Autodesk Fusion 360 part; units mm, degrees
(part 28 of 40)
  line L5956 (42.6094, 50.6358) -> (42.657, 50.79) construction
  line L5957 (42.657, 50.79) -> (42.7037, 50.9447) construction
  line L5958 (42.7037, 50.9447) -> (42.7495, 51.0999) construction
  line L5959 (42.7495, 51.0999) -> (42.7945, 51.2556) construction
  line L5960 (42.7945, 51.2556) -> (42.8386, 51.4118) construction
  line L5961 (42.8386, 51.4118) -> (42.8818, 51.5684) construction
  line L5962 (42.8818, 51.5684) -> (42.9241, 51.7255) construction
  line L5963 (42.9241, 51.7255) -> (42.9656, 51.883) construction
  line L5964 (42.9656, 51.883) -> (43.0063, 52.0409) construction
  line L5965 (43.0063, 52.0409) -> (43.0461, 52.1993) construction
  line L5966 (43.0461, 52.1993) -> (43.085, 52.3581) construction
  line L5967 (43.085, 52.3581) -> (43.1231, 52.5173) construction
  line L5968 (43.1231, 52.5173) -> (43.1604, 52.6769) construction
  line L5969 (43.1604, 52.6769) -> (43.1969, 52.8369) construction
  line L5970 (43.1969, 52.8369) -> (43.2326, 52.9973) construction
  line L5971 (43.2326, 52.9973) -> (43.2674, 53.1581) construction
  line L5972 (43.2674, 53.1581) -> (43.3015, 53.3193) construction
  line L5973 (43.3015, 53.3193) -> (43.3347, 53.4809) construction
  line L5974 (43.3347, 53.4809) -> (43.3672, 53.6428) construction
  line L5975 (43.3672, 53.6428) -> (43.3988, 53.8051) construction
  line L5976 (43.3988, 53.8051) -> (43.4297, 53.9677) construction
  line L5977 (43.4297, 53.9677) -> (43.4597, 54.1307) construction
  line L5978 (43.4597, 54.1307) -> (43.489, 54.294) construction
  line L5979 (43.489, 54.294) -> (43.5175, 54.4577) construction
  line L5980 (43.5175, 54.4577) -> (43.5453, 54.6217) construction
  line L5981 (43.5453, 54.6217) -> (43.5723, 54.7861) construction
  line L5982 (43.5723, 54.7861) -> (43.5984, 54.9508) construction
  line L5983 (43.5984, 54.9508) -> (43.6239, 55.1158) construction
  line L5984 (43.6239, 55.1158) -> (43.6486, 55.2811) construction
  line L5985 (43.6486, 55.2811) -> (43.6725, 55.4467) construction
  line L5986 (43.6725, 55.4467) -> (43.6956, 55.6126) construction
  line L5987 (43.6956, 55.6126) -> (43.718, 55.7789) construction
  line L5988 (43.718, 55.7789) -> (43.7397, 55.9454) construction
  line L5989 (43.7397, 55.9454) -> (43.7606, 56.1122) construction
  line L5990 (43.7606, 56.1122) -> (43.7767, 56.2459) construction
  line L5991 (43.7767, 56.2459) -> (43.7885, 56.3463) construction
  line L5992 (43.7885, 56.3463) -> (43.7962, 56.4133) construction
  line L5993 (43.7962, 56.4133) -> (43.8, 56.4469) construction
  arc A159 (-24.5301, 51.9354) -> (-27.5982, 50.3721) centre (0, 0) ccw
  arc A160 (-41.8132, -39.3784) -> (-39.3784, -41.8132) centre (0, 0) ccw
  line L5994 (-54.5366, 23.5481) -> (-56.0345, 24.1948)
  line L5995 (-57.9623, -13.005) -> (-59.5542, -13.3622)
  line L5996 (-44.5906, 39.2483) -> (-45.8153, 40.3263)
  line L5997 (13.005, 57.9623) -> (13.3622, 59.5542)
  line L5998 (51.1066, 30.2798) -> (52.5103, 31.1115)
  line L5999 (30.2798, -51.1066) -> (31.1115, -52.5103)
  arc A161 (41.8132, 39.3784) -> (39.3784, 41.8132) centre (0, 0) ccw
  line L6000 (157.5954, 173.5481) -> (156.0975, 174.1948)
  line L6001 (266.6686, 173.5481) -> (268.1665, 174.1948)
  line L6002 (271.2762, 155.5428) -> (272.9005, 155.6951)
  line L6003 (206.5892, 209.1442) -> (206.4369, 210.7685)
  line L6004 (199.127, 207.9623) -> (198.7698, 209.5542)
  line L6005 (251.3803, 194.5906) -> (252.4583, 195.8153)
  line L6006 (188.5839, 95.4634) -> (187.9372, 93.9655)
  arc A162 (157.5954, 173.5481) -> (160.1966, 174.5301) centre (158.3882, 175.3842) ccw
  arc A163 (160.1966, 125.4699) -> (157.5954, 126.4519) centre (158.3882, 124.6158) ccw
  arc A164 (251.5104, 108.1868) -> (251.3803, 105.4094) centre (252.8816, 106.7308) ccw
  arc A165 (262.5041, 122.4018) -> (263.2386, 119.7202) centre (264.2581, 121.4408) ccw
  spline S80 degree 5 poles (152.5778, 136.6378) (152.5477, 136.631) (152.4876, 136.6167) (152.3982, 136.5929) (152.2803, 136.5565) (152.1347, 136.5049) (151.9904, 136.4489) (151.8468, 136.3901) (151.7037, 136.3299) (151.5609, 136.2687) (151.4184, 136.2065) (151.2763, 136.1429) (151.1349, 136.0774) (150.9941, 136.0098) (150.8541, 135.94) (150.7147, 135.8684) (150.5759, 135.795) (150.4376, 135.7203) (150.2998, 135.6443) (150.1623, 135.5673) (150.0253, 135.4891) (149.8888, 135.4096) (149.7528, 135.3289) (149.6172, 135.247) (149.4822, 135.1637) (149.3477, 135.0792) (149.2136, 134.9936) (149.08, 134.9068) (148.9468, 134.819) (148.814, 134.7302) (148.6817, 134.6403) (148.5499, 134.5494) (148.4185, 134.4575) (148.2875, 134.3646) (148.157, 134.2707) (148.027, 134.1758) (147.8974, 134.08) (147.7682, 133.9832) (147.6394, 133.8854) (147.5111, 133.7868) (147.3832, 133.6873) (147.2558, 133.5869) (147.1288, 133.4856) (147.0022, 133.3834) (146.876, 133.2804) (146.7503, 133.1765) (146.625, 133.0717) (146.5002, 132.9662) (146.3758, 132.8598) (146.2518, 132.7526) (146.1282, 132.6445) (146.0051, 132.5357) (145.8823, 132.4261) (145.7601, 132.3158) (145.6382, 132.2046) (145.5168, 132.0927) (145.3958, 131.98) (145.2752, 131.8665) (145.1551, 131.7523) (145.0354, 131.6374) (144.9161, 131.5218) (144.7973, 131.4054) (144.6789, 131.2882) (144.5609, 131.1704) (144.4433, 131.0519) (144.3262, 130.9326) (144.2095, 130.8127) (144.0932, 130.6921) (143.9774, 130.5707) (143.862, 130.4488) (143.747, 130.3261) (143.6553, 130.2274) (143.5868, 130.1531) (143.5412, 130.1034) (143.5184, 130.0785) knots 0 0 0 0 0 0 0.01428571 0.02857143 0.04285714 0.05714286 0.07142857 0.08571429 0.1 0.11428571 0.12857143 0.14285714 0.15714286 0.17142857 0.18571429 0.2 0.21428571 0.22857143 0.24285714 0.25714286 0.27142857 0.28571429 0.3 0.31428571 0.32857143 0.34285714 0.35714286 0.37142857 0.38571429 0.4 0.41428571 0.42857143 0.44285714 0.45714286 0.47142857 0.48571429 0.5 0.51428571 0.52857143 0.54285714 0.55714286 0.57142857 0.58571429 0.6 0.61428571 0.62857143 0.64285714 0.65714286 0.67142857 0.68571429 0.7 0.71428571 0.72857143 0.74285714 0.75714286 0.77142857 0.78571429 0.8 0.81428571 0.82857143 0.84285714 0.85714286 0.87142857 0.88571429 0.9 0.91428571 0.92857143 0.94285714 0.95714286 0.97142857 0.98571429 1 1 1 1 1 1
  line L6007 (152.5778, 136.6378) -> (152.5477, 136.631) construction
  line L6008 (152.5477, 136.631) -> (152.4876, 136.6167) construction
  line L6009 (152.4876, 136.6167) -> (152.3982, 136.5929) construction
  line L6010 (152.3982, 136.5929) -> (152.2803, 136.5565) construction
  line L6011 (152.2803, 136.5565) -> (152.1347, 136.5049) construction
  line L6012 (152.1347, 136.5049) -> (151.9904, 136.4489) construction
  line L6013 (151.9904, 136.4489) -> (151.8468, 136.3901) construction
  line L6014 (151.8468, 136.3901) -> (151.7037, 136.3299) construction
  line L6015 (151.7037, 136.3299) -> (151.5609, 136.2687) construction
  line L6016 (151.5609, 136.2687) -> (151.4184, 136.2065) construction
  line L6017 (151.4184, 136.2065) -> (151.2763, 136.1429) construction
  line L6018 (151.2763, 136.1429) -> (151.1349, 136.0774) construction
  line L6019 (151.1349, 136.0774) -> (150.9941, 136.0098) construction
  line L6020 (150.9941, 136.0098) -> (150.8541, 135.94) construction
  line L6021 (150.8541, 135.94) -> (150.7147, 135.8684) construction
  line L6022 (150.7147, 135.8684) -> (150.5759, 135.795) construction
  line L6023 (150.5759, 135.795) -> (150.4376, 135.7203) construction
  line L6024 (150.4376, 135.7203) -> (150.2998, 135.6443) construction
  line L6025 (150.2998, 135.6443) -> (150.1623, 135.5673) construction
  line L6026 (150.1623, 135.5673) -> (150.0253, 135.4891) construction
  line L6027 (150.0253, 135.4891) -> (149.8888, 135.4096) construction
  line L6028 (149.8888, 135.4096) -> (149.7528, 135.3289) construction
  line L6029 (149.7528, 135.3289) -> (149.6172, 135.247) construction
  line L6030 (149.6172, 135.247) -> (149.4822, 135.1637) construction
  line L6031 (149.4822, 135.1637) -> (149.3477, 135.0792) construction
  line L6032 (149.3477, 135.0792) -> (149.2136, 134.9936) construction
  line L6033 (149.2136, 134.9936) -> (149.08, 134.9068) construction
  line L6034 (149.08, 134.9068) -> (148.9468, 134.819) construction
  line L6035 (148.9468, 134.819) -> (148.814, 134.7302) construction
  line L6036 (148.814, 134.7302) -> (148.6817, 134.6403) construction
  line L6037 (148.6817, 134.6403) -> (148.5499, 134.5494) construction
  line L6038 (148.5499, 134.5494) -> (148.4185, 134.4575) construction
  line L6039 (148.4185, 134.4575) -> (148.2875, 134.3646) construction
  line L6040 (148.2875, 134.3646) -> (148.157, 134.2707) construction
  line L6041 (148.157, 134.2707) -> (148.027, 134.1758) construction
  line L6042 (148.027, 134.1758) -> (147.8974, 134.08) construction
  line L6043 (147.8974, 134.08) -> (147.7682, 133.9832) construction
  line L6044 (147.7682, 133.9832) -> (147.6394, 133.8854) construction
  line L6045 (147.6394, 133.8854) -> (147.5111, 133.7868) construction
  line L6046 (147.5111, 133.7868) -> (147.3832, 133.6873) construction
  line L6047 (147.3832, 133.6873) -> (147.2558, 133.5869) construction
  line L6048 (147.2558, 133.5869) -> (147.1288, 133.4856) construction
  line L6049 (147.1288, 133.4856) -> (147.0022, 133.3834) construction
  line L6050 (147.0022, 133.3834) -> (146.876, 133.2804) construction
  line L6051 (146.876, 133.2804) -> (146.7503, 133.1765) construction
  line L6052 (146.7503, 133.1765) -> (146.625, 133.0717) construction
  line L6053 (146.625, 133.0717) -> (146.5002, 132.9662) construction
  line L6054 (146.5002, 132.9662) -> (146.3758, 132.8598) construction
  line L6055 (146.3758, 132.8598) -> (146.2518, 132.7526) construction
  line L6056 (146.2518, 132.7526) -> (146.1282, 132.6445) construction
  line L6057 (146.1282, 132.6445) -> (146.0051, 132.5357) construction
  line L6058 (146.0051, 132.5357) -> (145.8823, 132.4261) construction
  line L6059 (145.8823, 132.4261) -> (145.7601, 132.3158) construction
  line L6060 (145.7601, 132.3158) -> (145.6382, 132.2046) construction
  line L6061 (145.6382, 132.2046) -> (145.5168, 132.0927) construction
  line L6062 (145.5168, 132.0927) -> (145.3958, 131.98) construction
  line L6063 (145.3958, 131.98) -> (145.2752, 131.8665) construction
  line L6064 (145.2752, 131.8665) -> (145.1551, 131.7523) construction
  line L6065 (145.1551, 131.7523) -> (145.0354, 131.6374) construction
  line L6066 (145.0354, 131.6374) -> (144.9161, 131.5218) construction
  line L6067 (144.9161, 131.5218) -> (144.7973, 131.4054) construction
  line L6068 (144.7973, 131.4054) -> (144.6789, 131.2882) construction
  line L6069 (144.6789, 131.2882) -> (144.5609, 131.1704) construction
  line L6070 (144.5609, 131.1704) -> (144.4433, 131.0519) construction
  line L6071 (144.4433, 131.0519) -> (144.3262, 130.9326) construction
  line L6072 (144.3262, 130.9326) -> (144.2095, 130.8127) construction
  line L6073 (144.2095, 130.8127) -> (144.0932, 130.6921) construction
  line L6074 (144.0932, 130.6921) -> (143.9774, 130.5707) construction
  line L6075 (143.9774, 130.5707) -> (143.862, 130.4488) construction
  line L6076 (143.862, 130.4488) -> (143.747, 130.3261) construction
  line L6077 (143.747, 130.3261) -> (143.6553, 130.2274) construction
  line L6078 (143.6553, 130.2274) -> (143.5868, 130.1531) construction
  line L6079 (143.5868, 130.1531) -> (143.5412, 130.1034) construction
  line L6080 (143.5412, 130.1034) -> (143.5184, 130.0785) construction
  arc A166 (155.6851, 193.8) -> (153.0327, 190.1492) centre (212.132, 150) ccw
  spline S81 degree 5 poles (181.0205, 202.5103) (181.0048, 202.5368) (180.9726, 202.5895) (180.9223, 202.6672) (180.8513, 202.7681) (180.7572, 202.8906) (180.6593, 203.0106) (180.5591, 203.1289) (180.4576, 203.2464) (180.3553, 203.3634) (180.252, 203.4797) (180.1476, 203.5951) (180.0417, 203.7094) (179.9339, 203.8224) (179.8243, 203.934) (179.713, 204.0444) (179.6004, 204.1537) (179.4865, 204.2622) (179.3717, 204.3698) (179.256, 204.4767) (179.1393, 204.5828) (179.0215, 204.6881) (178.9028, 204.7926) (178.7829, 204.8961) (178.662, 204.9988) (178.5401, 205.1007) (178.4172, 205.2017) (178.2934, 205.302) (178.1687, 205.4015) (178.0432, 205.5003) (177.9169, 205.5984) (177.7897, 205.6957) (177.6617, 205.7923) (177.5329, 205.8881) (177.4032, 205.9832) (177.2728, 206.0776) (177.1415, 206.1712) (177.0096, 206.2642) (176.8768, 206.3564) (176.7434, 206.448) (176.6092, 206.5388) (176.4743, 206.629) (176.3387, 206.7185) (176.2025, 206.8073) (176.0655, 206.8955) (175.9278, 206.9829) (175.7895, 207.0697) (175.6505, 207.1558) (175.5109, 207.2413) (175.3706, 207.3261) (175.2297, 207.4102) (175.0882, 207.4937) (174.946, 207.5765) (174.8032, 207.6587) (174.6599, 207.7403) (174.5159, 207.8212) (174.3713, 207.9014) (174.2262, 207.981) (174.0805, 208.06) (173.9342, 208.1383) (173.7873, 208.216) (173.6399, 208.2931) (173.4919, 208.3695) (173.3434, 208.4453) (173.1943, 208.5205) (173.0447, 208.595) (172.8946, 208.669) (172.7439, 208.7423) (172.5927, 208.8149) (172.4411, 208.887) (172.2889, 208.9584) (172.1667, 209.0151) (172.0748, 209.0573) (172.0135, 209.0853) (171.9828, 209.0993) knots 0 0 0 0 0 0 0.01428571 0.02857143 0.04285714 0.05714286 0.07142857 0.08571429 0.1 0.11428571 0.12857143 0.14285714 0.15714286 0.17142857 0.18571429 0.2 0.21428571 0.22857143 0.24285714 0.25714286 0.27142857 0.28571429 0.3 0.31428571 0.32857143 0.34285714 0.35714286 0.37142857 0.38571429 0.4 0.41428571 0.42857143 0.44285714 0.45714286 0.47142857 0.48571429 0.5 0.51428571 0.52857143 0.54285714 0.55714286 0.57142857 0.58571429 0.6 0.61428571 0.62857143 0.64285714 0.65714286 0.67142857 0.68571429 0.7 0.71428571 0.72857143 0.74285714 0.75714286 0.77142857 0.78571429 0.8 0.81428571 0.82857143 0.84285714 0.85714286 0.87142857 0.88571429 0.9 0.91428571 0.92857143 0.94285714 0.95714286 0.97142857 0.98571429 1 1 1 1 1 1
  line L6081 (181.0205, 202.5103) -> (181.0048, 202.5368) construction
  line L6082 (181.0048, 202.5368) -> (180.9726, 202.5895) construction
  line L6083 (180.9726, 202.5895) -> (180.9223, 202.6672) construction
  line L6084 (180.9223, 202.6672) -> (180.8513, 202.7681) construction
  line L6085 (180.8513, 202.7681) -> (180.7572, 202.8906) construction
  line L6086 (180.7572, 202.8906) -> (180.6593, 203.0106) construction
  line L6087 (180.6593, 203.0106) -> (180.5591, 203.1289) construction
  line L6088 (180.5591, 203.1289) -> (180.4576, 203.2464) construction
  line L6089 (180.4576, 203.2464) -> (180.3553, 203.3634) construction
  line L6090 (180.3553, 203.3634) -> (180.252, 203.4797) construction
  line L6091 (180.252, 203.4797) -> (180.1476, 203.5951) construction
  line L6092 (180.1476, 203.5951) -> (180.0417, 203.7094) construction
  line L6093 (180.0417, 203.7094) -> (179.9339, 203.8224) construction
  line L6094 (179.9339, 203.8224) -> (179.8243, 203.934) construction
  line L6095 (179.8243, 203.934) -> (179.713, 204.0444) construction
  line L6096 (179.713, 204.0444) -> (179.6004, 204.1537) construction
  line L6097 (179.6004, 204.1537) -> (179.4865, 204.2622) construction
  line L6098 (179.4865, 204.2622) -> (179.3717, 204.3698) construction
  line L6099 (179.3717, 204.3698) -> (179.256, 204.4767) construction
  line L6100 (179.256, 204.4767) -> (179.1393, 204.5828) construction
  line L6101 (179.1393, 204.5828) -> (179.0215, 204.6881) construction
  line L6102 (179.0215, 204.6881) -> (178.9028, 204.7926) construction
  line L6103 (178.9028, 204.7926) -> (178.7829, 204.8961) construction
  line L6104 (178.7829, 204.8961) -> (178.662, 204.9988) construction
  line L6105 (178.662, 204.9988) -> (178.5401, 205.1007) construction
  line L6106 (178.5401, 205.1007) -> (178.4172, 205.2017) construction
  line L6107 (178.4172, 205.2017) -> (178.2934, 205.302) construction
  line L6108 (178.2934, 205.302) -> (178.1687, 205.4015) construction
  line L6109 (178.1687, 205.4015) -> (178.0432, 205.5003) construction
  line L6110 (178.0432, 205.5003) -> (177.9169, 205.5984) construction
  line L6111 (177.9169, 205.5984) -> (177.7897, 205.6957) construction
  line L6112 (177.7897, 205.6957) -> (177.6617, 205.7923) construction
  line L6113 (177.6617, 205.7923) -> (177.5329, 205.8881) construction
  line L6114 (177.5329, 205.8881) -> (177.4032, 205.9832) construction
  line L6115 (177.4032, 205.9832) -> (177.2728, 206.0776) construction
  line L6116 (177.2728, 206.0776) -> (177.1415, 206.1712) construction
  line L6117 (177.1415, 206.1712) -> (177.0096, 206.2642) construction
  line L6118 (177.0096, 206.2642) -> (176.8768, 206.3564) construction
  line L6119 (176.8768, 206.3564) -> (176.7434, 206.448) construction
  line L6120 (176.7434, 206.448) -> (176.6092, 206.5388) construction
  line L6121 (176.6092, 206.5388) -> (176.4743, 206.629) construction
  line L6122 (176.4743, 206.629) -> (176.3387, 206.7185) construction
  line L6123 (176.3387, 206.7185) -> (176.2025, 206.8073) construction
  line L6124 (176.2025, 206.8073) -> (176.0655, 206.8955) construction
  line L6125 (176.0655, 206.8955) -> (175.9278, 206.9829) construction
  line L6126 (175.9278, 206.9829) -> (175.7895, 207.0697) construction
  line L6127 (175.7895, 207.0697) -> (175.6505, 207.1558) construction
  line L6128 (175.6505, 207.1558) -> (175.5109, 207.2413) construction
  line L6129 (175.5109, 207.2413) -> (175.3706, 207.3261) construction
  line L6130 (175.3706, 207.3261) -> (175.2297, 207.4102) construction
  line L6131 (175.2297, 207.4102) -> (175.0882, 207.4937) construction
  line L6132 (175.0882, 207.4937) -> (174.946, 207.5765) construction
  line L6133 (174.946, 207.5765) -> (174.8032, 207.6587) construction
  line L6134 (174.8032, 207.6587) -> (174.6599, 207.7403) construction
  line L6135 (174.6599, 207.7403) -> (174.5159, 207.8212) construction
  line L6136 (174.5159, 207.8212) -> (174.3713, 207.9014) construction
  line L6137 (174.3713, 207.9014) -> (174.2262, 207.981) construction
  line L6138 (174.2262, 207.981) -> (174.0805, 208.06) construction
  line L6139 (174.0805, 208.06) -> (173.9342, 208.1383) construction
  line L6140 (173.9342, 208.1383) -> (173.7873, 208.216) construction
  line L6141 (173.7873, 208.216) -> (173.6399, 208.2931) construction
  line L6142 (173.6399, 208.2931) -> (173.4919, 208.3695) construction
  line L6143 (173.4919, 208.3695) -> (173.3434, 208.4453) construction
  line L6144 (173.3434, 208.4453) -> (173.1943, 208.5205) construction
  line L6145 (173.1943, 208.5205) -> (173.0447, 208.595) construction
  line L6146 (173.0447, 208.595) -> (172.8946, 208.669) construction
  line L6147 (172.8946, 208.669) -> (172.7439, 208.7423) construction
  line L6148 (172.7439, 208.7423) -> (172.5927, 208.8149) construction
  line L6149 (172.5927, 208.8149) -> (172.4411, 208.887) construction
  line L6150 (172.4411, 208.887) -> (172.2889, 208.9584) construction
  line L6151 (172.2889, 208.9584) -> (172.1667, 209.0151) construction
  line L6152 (172.1667, 209.0151) -> (172.0748, 209.0573) construction
  line L6153 (172.0748, 209.0573) -> (172.0135, 209.0853) construction
  line L6154 (172.0135, 209.0853) -> (171.9828, 209.0993) construction
  spline S82 degree 5 poles (198.7698, 209.5542) (198.763, 209.5843) (198.7487, 209.6444) (198.7249, 209.7338) (198.6885, 209.8517) (198.6369, 209.9973) (198.5809, 210.1416) (198.5221, 210.2852) (198.4619, 210.4283) (198.4007, 210.5711) (198.3385, 210.7136) (198.2749, 210.8557) (198.2094, 210.9971) (198.1418, 211.1379) (198.072, 211.2779) (198.0004, 211.4173) (197.927, 211.5561) (197.8523, 211.6944) (197.7763, 211.8322) (197.6993, 211.9697) (197.6211, 212.1067) (197.5416, 212.2432) (197.4609, 212.3792) (197.379, 212.5148) (197.2957, 212.6498) (197.2112, 212.7843) (197.1256, 212.9184) (197.0388, 213.052) (196.951, 213.1852) (196.8622, 213.318) (196.7723, 213.4503) (196.6814, 213.5821) (196.5895, 213.7135) (196.4966, 213.8445) (196.4027, 213.975) (196.3078, 214.105) (196.212, 214.2346) (196.1152, 214.3638) (196.0174, 214.4926) (195.9188, 214.6209) (195.8193, 214.7488) (195.7189, 214.8762) (195.6176, 215.0032) (195.5154, 215.1298) (195.4124, 215.256) (195.3085, 215.3817) (195.2037, 215.507) (195.0982, 215.6318) (194.9918, 215.7562) (194.8846, 215.8802) (194.7765, 216.0038) (194.6677, 216.1269) (194.5581, 216.2497) (194.4478, 216.3719) (194.3366, 216.4938) (194.2247, 216.6152) (194.112, 216.7362) (193.9985, 216.8568) (193.8843, 216.9769) (193.7694, 217.0966) (193.6538, 217.2159) (193.5374, 217.3347) (193.4202, 217.4531) (193.3024, 217.5711) (193.1839, 217.6887) (193.0646, 217.8058) (192.9447, 217.9225) (192.8241, 218.0388) (192.7027, 218.1546) (192.5808, 218.27) (192.4581, 218.385) (192.3594, 218.4767) (192.2851, 218.5452) (192.2354, 218.5908) (192.2105, 218.6136) knots 0 0 0 0 0 0 0.01428571 0.02857143 0.04285714 0.05714286 0.07142857 0.08571429 0.1 0.11428571 0.12857143 0.14285714 0.15714286 0.17142857 0.18571429 0.2 0.21428571 0.22857143 0.24285714 0.25714286 0.27142857 0.28571429 0.3 0.31428571 0.32857143 0.34285714 0.35714286 0.37142857 0.38571429 0.4 0.41428571 0.42857143 0.44285714 0.45714286 0.47142857 0.48571429 0.5 0.51428571 0.52857143 0.54285714 0.55714286 0.57142857 0.58571429 0.6 0.61428571 0.62857143 0.64285714 0.65714286 0.67142857 0.68571429 0.7 0.71428571 0.72857143 0.74285714 0.75714286 0.77142857 0.78571429 0.8 0.81428571 0.82857143 0.84285714 0.85714286 0.87142857 0.88571429 0.9 0.91428571 0.92857143 0.94285714 0.95714286 0.97142857 0.98571429 1 1 1 1 1 1
  line L6155 (198.7698, 209.5542) -> (198.763, 209.5843) construction
  line L6156 (198.763, 209.5843) -> (198.7487, 209.6444) construction
  line L6157 (198.7487, 209.6444) -> (198.7249, 209.7338) construction
  line L6158 (198.7249, 209.7338) -> (198.6885, 209.8517) construction
  line L6159 (198.6885, 209.8517) -> (198.6369, 209.9973) construction
  line L6160 (198.6369, 209.9973) -> (198.5809, 210.1416) construction
  line L6161 (198.5809, 210.1416) -> (198.5221, 210.2852) construction
  line L6162 (198.5221, 210.2852) -> (198.4619, 210.4283) construction
  line L6163 (198.4619, 210.4283) -> (198.4007, 210.5711) construction
  line L6164 (198.4007, 210.5711) -> (198.3385, 210.7136) construction
  line L6165 (198.3385, 210.7136) -> (198.2749, 210.8557) construction
  line L6166 (198.2749, 210.8557) -> (198.2094, 210.9971) construction
  line L6167 (198.2094, 210.9971) -> (198.1418, 211.1379) construction
  line L6168 (198.1418, 211.1379) -> (198.072, 211.2779) construction
  line L6169 (198.072, 211.2779) -> (198.0004, 211.4173) construction
  line L6170 (198.0004, 211.4173) -> (197.927, 211.5561) construction
  line L6171 (197.927, 211.5561) -> (197.8523, 211.6944) construction
  line L6172 (197.8523, 211.6944) -> (197.7763, 211.8322) construction
  line L6173 (197.7763, 211.8322) -> (197.6993, 211.9697) construction
  line L6174 (197.6993, 211.9697) -> (197.6211, 212.1067) construction
  line L6175 (197.6211, 212.1067) -> (197.5416, 212.2432) construction
  line L6176 (197.5416, 212.2432) -> (197.4609, 212.3792) construction
  line L6177 (197.4609, 212.3792) -> (197.379, 212.5148) construction
  line L6178 (197.379, 212.5148) -> (197.2957, 212.6498) construction
  line L6179 (197.2957, 212.6498) -> (197.2112, 212.7843) construction
  line L6180 (197.2112, 212.7843) -> (197.1256, 212.9184) construction
  line L6181 (197.1256, 212.9184) -> (197.0388, 213.052) construction
  line L6182 (197.0388, 213.052) -> (196.951, 213.1852) construction
  line L6183 (196.951, 213.1852) -> (196.8622, 213.318) construction
  line L6184 (196.8622, 213.318) -> (196.7723, 213.4503) construction
  line L6185 (196.7723, 213.4503) -> (196.6814, 213.5821) construction
  line L6186 (196.6814, 213.5821) -> (196.5895, 213.7135) construction
  line L6187 (196.5895, 213.7135) -> (196.4966, 213.8445) construction
  line L6188 (196.4966, 213.8445) -> (196.4027, 213.975) construction
  line L6189 (196.4027, 213.975) -> (196.3078, 214.105) construction
  line L6190 (196.3078, 214.105) -> (196.212, 214.2346) construction
  line L6191 (196.212, 214.2346) -> (196.1152, 214.3638) construction
  line L6192 (196.1152, 214.3638) -> (196.0174, 214.4926) construction
  line L6193 (196.0174, 214.4926) -> (195.9188, 214.6209) construction
  line L6194 (195.9188, 214.6209) -> (195.8193, 214.7488) construction
  line L6195 (195.8193, 214.7488) -> (195.7189, 214.8762) construction
  line L6196 (195.7189, 214.8762) -> (195.6176, 215.0032) construction
  line L6197 (195.6176, 215.0032) -> (195.5154, 215.1298) construction
  line L6198 (195.5154, 215.1298) -> (195.4124, 215.256) construction
  line L6199 (195.4124, 215.256) -> (195.3085, 215.3817) construction
  line L6200 (195.3085, 215.3817) -> (195.2037, 215.507) construction
  line L6201 (195.2037, 215.507) -> (195.0982, 215.6318) construction
  line L6202 (195.0982, 215.6318) -> (194.9918, 215.7562) construction
  line L6203 (194.9918, 215.7562) -> (194.8846, 215.8802) construction
  line L6204 (194.8846, 215.8802) -> (194.7765, 216.0038) construction
  line L6205 (194.7765, 216.0038) -> (194.6677, 216.1269) construction
  line L6206 (194.6677, 216.1269) -> (194.5581, 216.2497) construction
  line L6207 (194.5581, 216.2497) -> (194.4478, 216.3719) construction
  line L6208 (194.4478, 216.3719) -> (194.3366, 216.4938) construction
  line L6209 (194.3366, 216.4938) -> (194.2247, 216.6152) construction
  line L6210 (194.2247, 216.6152) -> (194.112, 216.7362) construction
  line L6211 (194.112, 216.7362) -> (193.9985, 216.8568) construction
  line L6212 (193.9985, 216.8568) -> (193.8843, 216.9769) construction
  line L6213 (193.8843, 216.9769) -> (193.7694, 217.0966) construction
  line L6214 (193.7694, 217.0966) -> (193.6538, 217.2159) construction
  line L6215 (193.6538, 217.2159) -> (193.5374, 217.3347) construction
  line L6216 (193.5374, 217.3347) -> (193.4202, 217.4531) construction
  line L6217 (193.4202, 217.4531) -> (193.3024, 217.5711) construction
  line L6218 (193.3024, 217.5711) -> (193.1839, 217.6887) construction
  line L6219 (193.1839, 217.6887) -> (193.0646, 217.8058) construction
  line L6220 (193.0646, 217.8058) -> (192.9447, 217.9225) construction
  line L6221 (192.9447, 217.9225) -> (192.8241, 218.0388) construction
  line L6222 (192.8241, 218.0388) -> (192.7027, 218.1546) construction
  line L6223 (192.7027, 218.1546) -> (192.5808, 218.27) construction
  line L6224 (192.5808, 218.27) -> (192.4581, 218.385) construction
  line L6225 (192.4581, 218.385) -> (192.3594, 218.4767) construction
  line L6226 (192.3594, 218.4767) -> (192.2851, 218.5452) construction
  line L6227 (192.2851, 218.5452) -> (192.2354, 218.5908) construction
  line L6228 (192.2354, 218.5908) -> (192.2105, 218.6136) construction
  arc A167 (255.932, 206.4469) -> (252.2812, 209.0993) centre (212.132, 150) ccw
  arc A168 (271.2313, 190.1492) -> (268.5789, 193.8) centre (212.132, 150) ccw
  spline S83 degree 5 poles (272.9005, 155.6951) (272.9313, 155.6979) (272.9929, 155.7029) (273.0853, 155.7078) (273.2086, 155.7097) (273.363, 155.7056) (273.5176, 155.6969) (273.6723, 155.6854) (273.827, 155.6723) (273.9818, 155.6583) (274.1365, 155.6431) (274.2913, 155.6265) (274.446, 155.608) (274.6008, 155.5871) (274.7555, 155.5641) (274.9102, 155.539) (275.0649, 155.5121) (275.2195, 155.4838) (275.3741, 155.4542) (275.5286, 155.4233) (275.6831, 155.3913) (275.8375, 155.3579) (275.9918, 155.3232) (276.146, 155.2871) (276.3002, 155.2497) (276.4542, 155.2109) (276.6082, 155.1709) (276.7621, 155.1297) (276.9159, 155.0873) (277.0696, 155.0439) (277.2232, 154.9993) (277.3767, 154.9536) (277.53, 154.9068) (277.6833, 154.8589) (277.8364, 154.8099) (277.9894, 154.7599) (278.1423, 154.7087) (278.2951, 154.6566) (278.4478, 154.6035) (278.6003, 154.5493) (278.7526, 154.4942) (278.9049, 154.438) (279.057, 154.381) (279.209, 154.3229) (279.3608, 154.2639) (279.5124, 154.2039) (279.664, 154.143) (279.8153, 154.0812) (279.9665, 154.0185) (280.1176, 153.9548) (280.2685, 153.8903) (280.4192, 153.8249) (280.5698, 153.7585) (280.7202, 153.6913) (280.8704, 153.6233) (281.0205, 153.5543) (281.1704, 153.4846) (281.3201, 153.4139) (281.4696, 153.3425) (281.619, 153.2701) (281.7682, 153.197) (281.9172, 153.123) (282.066, 153.0482) (282.2146, 152.9726) (282.3631, 152.8962) (282.5113, 152.819) (282.6594, 152.741) (282.8072, 152.6622) (282.9549, 152.5826) (283.1023, 152.5023) (283.2496, 152.4211) (283.3672, 152.3556) (283.4554, 152.3061) (283.5141, 152.2729) (283.5435, 152.2563) knots 0 0 0 0 0 0 0.01428571 0.02857143 0.04285714 0.05714286 0.07142857 0.08571429 0.1 0.11428571 0.12857143 0.14285714 0.15714286 0.17142857 0.18571429 0.2 0.21428571 0.22857143 0.24285714 0.25714286 0.27142857 0.28571429 0.3 0.31428571 0.32857143 0.34285714 0.35714286 0.37142857 0.38571429 0.4 0.41428571 0.42857143 0.44285714 0.45714286 0.47142857 0.48571429 0.5 0.51428571 0.52857143 0.54285714 0.55714286 0.57142857 0.58571429 0.6 0.61428571 0.62857143 0.64285714 0.65714286 0.67142857 0.68571429 0.7 0.71428571 0.72857143 0.74285714 0.75714286 0.77142857 0.78571429 0.8 0.81428571 0.82857143 0.84285714 0.85714286 0.87142857 0.88571429 0.9 0.91428571 0.92857143 0.94285714 0.95714286 0.97142857 0.98571429 1 1 1 1 1 1
  line L6229 (272.9005, 155.6951) -> (272.9313, 155.6979) construction
  line L6230 (272.9313, 155.6979) -> (272.9929, 155.7029) construction
  line L6231 (272.9929, 155.7029) -> (273.0853, 155.7078) construction
  line L6232 (273.0853, 155.7078) -> (273.2086, 155.7097) construction
  line L6233 (273.2086, 155.7097) -> (273.363, 155.7056) construction
  line L6234 (273.363, 155.7056) -> (273.5176, 155.6969) construction
  line L6235 (273.5176, 155.6969) -> (273.6723, 155.6854) construction
  line L6236 (273.6723, 155.6854) -> (273.827, 155.6723) construction
  line L6237 (273.827, 155.6723) -> (273.9818, 155.6583) construction
  line L6238 (273.9818, 155.6583) -> (274.1365, 155.6431) construction
  line L6239 (274.1365, 155.6431) -> (274.2913, 155.6265) construction
  line L6240 (274.2913, 155.6265) -> (274.446, 155.608) construction
  line L6241 (274.446, 155.608) -> (274.6008, 155.5871) construction
  line L6242 (274.6008, 155.5871) -> (274.7555, 155.5641) construction
  line L6243 (274.7555, 155.5641) -> (274.9102, 155.539) construction
  line L6244 (274.9102, 155.539) -> (275.0649, 155.5121) construction
  line L6245 (275.0649, 155.5121) -> (275.2195, 155.4838) construction
  line L6246 (275.2195, 155.4838) -> (275.3741, 155.4542) construction
  line L6247 (275.3741, 155.4542) -> (275.5286, 155.4233) construction
  line L6248 (275.5286, 155.4233) -> (275.6831, 155.3913) construction
  line L6249 (275.6831, 155.3913) -> (275.8375, 155.3579) construction
  line L6250 (275.8375, 155.3579) -> (275.9918, 155.3232) construction
  line L6251 (275.9918, 155.3232) -> (276.146, 155.2871) construction
  line L6252 (276.146, 155.2871) -> (276.3002, 155.2497) construction
  line L6253 (276.3002, 155.2497) -> (276.4542, 155.2109) construction
  line L6254 (276.4542, 155.2109) -> (276.6082, 155.1709) construction
  line L6255 (276.6082, 155.1709) -> (276.7621, 155.1297) construction
  line L6256 (276.7621, 155.1297) -> (276.9159, 155.0873) construction
  line L6257 (276.9159, 155.0873) -> (277.0696, 155.0439) construction
  line L6258 (277.0696, 155.0439) -> (277.2232, 154.9993) construction
  line L6259 (277.2232, 154.9993) -> (277.3767, 154.9536) construction
  line L6260 (277.3767, 154.9536) -> (277.53, 154.9068) construction
  line L6261 (277.53, 154.9068) -> (277.6833, 154.8589) construction
  line L6262 (277.6833, 154.8589) -> (277.8364, 154.8099) construction
  line L6263 (277.8364, 154.8099) -> (277.9894, 154.7599) construction
  line L6264 (277.9894, 154.7599) -> (278.1423, 154.7087) construction
  line L6265 (278.1423, 154.7087) -> (278.2951, 154.6566) construction
  line L6266 (278.2951, 154.6566) -> (278.4478, 154.6035) construction
  line L6267 (278.4478, 154.6035) -> (278.6003, 154.5493) construction
  line L6268 (278.6003, 154.5493) -> (278.7526, 154.4942) construction
  line L6269 (278.7526, 154.4942) -> (278.9049, 154.438) construction
  line L6270 (278.9049, 154.438) -> (279.057, 154.381) construction
  line L6271 (279.057, 154.381) -> (279.209, 154.3229) construction
  line L6272 (279.209, 154.3229) -> (279.3608, 154.2639) construction
  line L6273 (279.3608, 154.2639) -> (279.5124, 154.2039) construction
  line L6274 (279.5124, 154.2039) -> (279.664, 154.143) construction
  line L6275 (279.664, 154.143) -> (279.8153, 154.0812) construction
  line L6276 (279.8153, 154.0812) -> (279.9665, 154.0185) construction
  line L6277 (279.9665, 154.0185) -> (280.1176, 153.9548) construction
  line L6278 (280.1176, 153.9548) -> (280.2685, 153.8903) construction
  line L6279 (280.2685, 153.8903) -> (280.4192, 153.8249) construction
  line L6280 (280.4192, 153.8249) -> (280.5698, 153.7585) construction
  line L6281 (280.5698, 153.7585) -> (280.7202, 153.6913) construction
  line L6282 (280.7202, 153.6913) -> (280.8704, 153.6233) construction
  line L6283 (280.8704, 153.6233) -> (281.0205, 153.5543) construction
  line L6284 (281.0205, 153.5543) -> (281.1704, 153.4846) construction
  line L6285 (281.1704, 153.4846) -> (281.3201, 153.4139) construction
  line L6286 (281.3201, 153.4139) -> (281.4696, 153.3425) construction
  line L6287 (281.4696, 153.3425) -> (281.619, 153.2701) construction
  line L6288 (281.619, 153.2701) -> (281.7682, 153.197) construction
  line L6289 (281.7682, 153.197) -> (281.9172, 153.123) construction
  line L6290 (281.9172, 153.123) -> (282.066, 153.0482) construction
  line L6291 (282.066, 153.0482) -> (282.2146, 152.9726) construction
  line L6292 (282.2146, 152.9726) -> (282.3631, 152.8962) construction
  line L6293 (282.3631, 152.8962) -> (282.5113, 152.819) construction
  line L6294 (282.5113, 152.819) -> (282.6594, 152.741) construction
  line L6295 (282.6594, 152.741) -> (282.8072, 152.6622) construction
  line L6296 (282.8072, 152.6622) -> (282.9549, 152.5826) construction
  line L6297 (282.9549, 152.5826) -> (283.1023, 152.5023) construction
  line L6298 (283.1023, 152.5023) -> (283.2496, 152.4211) construction
  line L6299 (283.2496, 152.4211) -> (283.3672, 152.3556) construction
  line L6300 (283.3672, 152.3556) -> (283.4554, 152.3061) construction
  line L6301 (283.4554, 152.3061) -> (283.5141, 152.2729) construction
  line L6302 (283.5141, 152.2729) -> (283.5435, 152.2563) construction
  arc A169 (262.5041, 122.4018) -> (264.0674, 125.4699) centre (212.132, 150) ccw
  arc A170 (279.3511, 125.7868) -> (280.7456, 130.0785) centre (212.132, 150) ccw
  spline S84 degree 5 poles (159.6217, 118.8885) (159.5952, 118.8728) (159.5425, 118.8406) (159.4648, 118.7903) (159.3639, 118.7193) (159.2414, 118.6252) (159.1214, 118.5273) (159.0031, 118.4271) (158.8856, 118.3256) (158.7686, 118.2233) (158.6523, 118.12) (158.5369, 118.0156) (158.4226, 117.9097) (158.3096, 117.8019) (158.198, 117.6923) (158.0876, 117.581) (157.9783, 117.4684) (157.8698, 117.3545) (157.7622, 117.2397) (157.6553, 117.124) (157.5492, 117.0073) (157.4439, 116.8895) (157.3394, 116.7708) (157.2359, 116.6509) (157.1332, 116.53) (157.0313, 116.4081) (156.9303, 116.2852) (156.83, 116.1614) (156.7305, 116.0367) (156.6317, 115.9112) (156.5336, 115.7849) (156.4363, 115.6577) (156.3397, 115.5297) (156.2439, 115.4009) (156.1488, 115.2712) (156.0544, 115.1408) (155.9608, 115.0095) (155.8678, 114.8776) (155.7756, 114.7448) (155.684, 114.6114) (155.5932, 114.4772) (155.503, 114.3423) (155.4135, 114.2067) (155.3247, 114.0705) (155.2365, 113.9335) (155.1491, 113.7958) (155.0623, 113.6575) (154.9762, 113.5185) (154.8907, 113.3789) (154.8059, 113.2386) (154.7218, 113.0977) (154.6383, 112.9562) (154.5555, 112.814) (154.4733, 112.6712) (154.3917, 112.5279) (154.3108, 112.3839) (154.2306, 112.2393) (154.151, 112.0942) (154.072, 111.9485) (153.9937, 111.8022) (153.916, 111.6553) (153.8389, 111.5079) (153.7625, 111.3599) (153.6867, 111.2114) (153.6115, 111.0623) (153.537, 110.9127) (153.463, 110.7626) (153.3897, 110.6119) (153.3171, 110.4607) (153.245, 110.3091) (153.1736, 110.1569) (153.1169, 110.0347) (153.0747, 109.9428) (153.0467, 109.8815) (153.0327, 109.8508) knots 0 0 0 0 0 0 0.01428571 0.02857143 0.04285714 0.05714286 0.07142857 0.08571429 0.1 0.11428571 0.12857143 0.14285714 0.15714286 0.17142857 0.18571429 0.2 0.21428571 0.22857143 0.24285714 0.25714286 0.27142857 0.28571429 0.3 0.31428571 0.32857143 0.34285714 0.35714286 0.37142857 0.38571429 0.4 0.41428571 0.42857143 0.44285714 0.45714286 0.47142857 0.48571429 0.5 0.51428571 0.52857143 0.54285714 0.55714286 0.57142857 0.58571429 0.6 0.61428571 0.62857143 0.64285714 0.65714286 0.67142857 0.68571429 0.7 0.71428571 0.72857143 0.74285714 0.75714286 0.77142857 0.78571429 0.8 0.81428571 0.82857143 0.84285714 0.85714286 0.87142857 0.88571429 0.9 0.91428571 0.92857143 0.94285714 0.95714286 0.97142857 0.98571429 1 1 1 1 1 1
  line L6303 (159.6217, 118.8885) -> (159.5952, 118.8728) construction
  line L6304 (159.5952, 118.8728) -> (159.5425, 118.8406) construction
  line L6305 (159.5425, 118.8406) -> (159.4648, 118.7903) construction
  line L6306 (159.4648, 118.7903) -> (159.3639, 118.7193) construction
  line L6307 (159.3639, 118.7193) -> (159.2414, 118.6252) construction
  line L6308 (159.2414, 118.6252) -> (159.1214, 118.5273) construction
  line L6309 (159.1214, 118.5273) -> (159.0031, 118.4271) construction
  line L6310 (159.0031, 118.4271) -> (158.8856, 118.3256) construction
  line L6311 (158.8856, 118.3256) -> (158.7686, 118.2233) construction
  line L6312 (158.7686, 118.2233) -> (158.6523, 118.12) construction
  line L6313 (158.6523, 118.12) -> (158.5369, 118.0156) construction
  line L6314 (158.5369, 118.0156) -> (158.4226, 117.9097) construction
  line L6315 (158.4226, 117.9097) -> (158.3096, 117.8019) construction
  line L6316 (158.3096, 117.8019) -> (158.198, 117.6923) construction
  line L6317 (158.198, 117.6923) -> (158.0876, 117.581) construction
  line L6318 (158.0876, 117.581) -> (157.9783, 117.4684) construction
  line L6319 (157.9783, 117.4684) -> (157.8698, 117.3545) construction
  line L6320 (157.8698, 117.3545) -> (157.7622, 117.2397) construction
  line L6321 (157.7622, 117.2397) -> (157.6553, 117.124) construction
  line L6322 (157.6553, 117.124) -> (157.5492, 117.0073) construction
  line L6323 (157.5492, 117.0073) -> (157.4439, 116.8895) construction
  line L6324 (157.4439, 116.8895) -> (157.3394, 116.7708) construction
  line L6325 (157.3394, 116.7708) -> (157.2359, 116.6509) construction
  line L6326 (157.2359, 116.6509) -> (157.1332, 116.53) construction
  line L6327 (157.1332, 116.53) -> (157.0313, 116.4081) construction
  line L6328 (157.0313, 116.4081) -> (156.9303, 116.2852) construction
  line L6329 (156.9303, 116.2852) -> (156.83, 116.1614) construction
  line L6330 (156.83, 116.1614) -> (156.7305, 116.0367) construction
  line L6331 (156.7305, 116.0367) -> (156.6317, 115.9112) construction
  line L6332 (156.6317, 115.9112) -> (156.5336, 115.7849) construction
  line L6333 (156.5336, 115.7849) -> (156.4363, 115.6577) construction
  line L6334 (156.4363, 115.6577) -> (156.3397, 115.5297) construction
  line L6335 (156.3397, 115.5297) -> (156.2439, 115.4009) construction
  line L6336 (156.2439, 115.4009) -> (156.1488, 115.2712) construction
  line L6337 (156.1488, 115.2712) -> (156.0544, 115.1408) construction
  line L6338 (156.0544, 115.1408) -> (155.9608, 115.0095) construction
  line L6339 (155.9608, 115.0095) -> (155.8678, 114.8776) construction
  line L6340 (155.8678, 114.8776) -> (155.7756, 114.7448) construction
  line L6341 (155.7756, 114.7448) -> (155.684, 114.6114) construction
  line L6342 (155.684, 114.6114) -> (155.5932, 114.4772) construction
  line L6343 (155.5932, 114.4772) -> (155.503, 114.3423) construction
  line L6344 (155.503, 114.3423) -> (155.4135, 114.2067) construction
  line L6345 (155.4135, 114.2067) -> (155.3247, 114.0705) construction
  line L6346 (155.3247, 114.0705) -> (155.2365, 113.9335) construction
  line L6347 (155.2365, 113.9335) -> (155.1491, 113.7958) construction
  line L6348 (155.1491, 113.7958) -> (155.0623, 113.6575) construction
  line L6349 (155.0623, 113.6575) -> (154.9762, 113.5185) construction
  line L6350 (154.9762, 113.5185) -> (154.8907, 113.3789) construction
  line L6351 (154.8907, 113.3789) -> (154.8059, 113.2386) construction
  line L6352 (154.8059, 113.2386) -> (154.7218, 113.0977) construction
  line L6353 (154.7218, 113.0977) -> (154.6383, 112.9562) construction
  line L6354 (154.6383, 112.9562) -> (154.5555, 112.814) construction
  line L6355 (154.5555, 112.814) -> (154.4733, 112.6712) construction
  line L6356 (154.4733, 112.6712) -> (154.3917, 112.5279) construction
  line L6357 (154.3917, 112.5279) -> (154.3108, 112.3839) construction
  line L6358 (154.3108, 112.3839) -> (154.2306, 112.2393) construction
  line L6359 (154.2306, 112.2393) -> (154.151, 112.0942) construction
  line L6360 (154.151, 112.0942) -> (154.072, 111.9485) construction
  line L6361 (154.072, 111.9485) -> (153.9937, 111.8022) construction
  line L6362 (153.9937, 111.8022) -> (153.916, 111.6553) construction
  line L6363 (153.916, 111.6553) -> (153.8389, 111.5079) construction
  line L6364 (153.8389, 111.5079) -> (153.7625, 111.3599) construction
  line L6365 (153.7625, 111.3599) -> (153.6867, 111.2114) construction
  line L6366 (153.6867, 111.2114) -> (153.6115, 111.0623) construction
  line L6367 (153.6115, 111.0623) -> (153.537, 110.9127) construction
  line L6368 (153.537, 110.9127) -> (153.463, 110.7626) construction
  line L6369 (153.463, 110.7626) -> (153.3897, 110.6119) construction
  line L6370 (153.3897, 110.6119) -> (153.3171, 110.4607) construction
  line L6371 (153.3171, 110.4607) -> (153.245, 110.3091) construction
  line L6372 (153.245, 110.3091) -> (153.1736, 110.1569) construction
  line L6373 (153.1736, 110.1569) -> (153.1169, 110.0347) construction
  line L6374 (153.1169, 110.0347) -> (153.0747, 109.9428) construction
  line L6375 (153.0747, 109.9428) -> (153.0467, 109.8815) construction
  line L6376 (153.0467, 109.8815) -> (153.0327, 109.8508) construction
  spline S85 degree 5 poles (272.9005, 144.3049) (272.9313, 144.3021) (272.9929, 144.2971) (273.0853, 144.2922) (273.2086, 144.2903) (273.363, 144.2944) (273.5176, 144.3031) (273.6723, 144.3146) (273.827, 144.3277) (273.9818, 144.3417) (274.1365, 144.3569) (274.2913, 144.3735) (274.446, 144.392) (274.6008, 144.4129) (274.7555, 144.4359) (274.9102, 144.461) (275.0649, 144.4879) (275.2195, 144.5162) (275.3741, 144.5458) (275.5286, 144.5767) (275.6831, 144.6087) (275.8375, 144.6421) (275.9918, 144.6768) (276.146, 144.7129) (276.3002, 144.7503) (276.4542, 144.7891) (276.6082, 144.8291) (276.7621, 144.8703) (276.9159, 144.9127) (277.0696, 144.9561) (277.2232, 145.0007) (277.3767, 145.0464) (277.53, 145.0932) (277.6833, 145.1411) (277.8364, 145.1901) (277.9894, 145.2401) (278.1423, 145.2913) (278.2951, 145.3434) (278.4478, 145.3965) (278.6003, 145.4507) (278.7526, 145.5058) (278.9049, 145.562) (279.057, 145.619) (279.209, 145.6771) (279.3608, 145.7361) (279.5124, 145.7961) (279.664, 145.857) (279.8153, 145.9188) (279.9665, 145.9815) (280.1176, 146.0452) (280.2685, 146.1097) (280.4192, 146.1751) (280.5698, 146.2415) (280.7202, 146.3087) (280.8704, 146.3767) (281.0205, 146.4457) (281.1704, 146.5154) (281.3201, 146.5861) (281.4696, 146.6575) (281.619, 146.7299) (281.7682, 146.803) (281.9172, 146.877) (282.066, 146.9518) (282.2146, 147.0274) (282.3631, 147.1038) (282.5113, 147.181) (282.6594, 147.259) (282.8072, 147.3378) (282.9549, 147.4174) (283.1023, 147.4977) (283.2496, 147.5789) (283.3672, 147.6444) (283.4554, 147.6939) (283.5141, 147.7271) (283.5435, 147.7437) knots 0 0 0 0 0 0 0.01428571 0.02857143 0.04285714 0.05714286 0.07142857 0.08571429 0.1 0.11428571 0.12857143 0.14285714 0.15714286 0.17142857 0.18571429 0.2 0.21428571 0.22857143 0.24285714 0.25714286 0.27142857 0.28571429 0.3 0.31428571 0.32857143 0.34285714 0.35714286 0.37142857 0.38571429 0.4 0.41428571 0.42857143 0.44285714 0.45714286 0.47142857 0.48571429 0.5 0.51428571 0.52857143 0.54285714 0.55714286 0.57142857 0.58571429 0.6 0.61428571 0.62857143 0.64285714 0.65714286 0.67142857 0.68571429 0.7 0.71428571 0.72857143 0.74285714 0.75714286 0.77142857 0.78571429 0.8 0.81428571 0.82857143 0.84285714 0.85714286 0.87142857 0.88571429 0.9 0.91428571 0.92857143 0.94285714 0.95714286 0.97142857 0.98571429 1 1 1 1 1 1
  line L6377 (272.9005, 144.3049) -> (272.9313, 144.3021) construction
  line L6378 (272.9313, 144.3021) -> (272.9929, 144.2971) construction
  line L6379 (272.9929, 144.2971) -> (273.0853, 144.2922) construction
  line L6380 (273.0853, 144.2922) -> (273.2086, 144.2903) construction
  line L6381 (273.2086, 144.2903) -> (273.363, 144.2944) construction
  line L6382 (273.363, 144.2944) -> (273.5176, 144.3031) construction
  line L6383 (273.5176, 144.3031) -> (273.6723, 144.3146) construction
  line L6384 (273.6723, 144.3146) -> (273.827, 144.3277) construction
  line L6385 (273.827, 144.3277) -> (273.9818, 144.3417) construction
  line L6386 (273.9818, 144.3417) -> (274.1365, 144.3569) construction
  line L6387 (274.1365, 144.3569) -> (274.2913, 144.3735) construction
  line L6388 (274.2913, 144.3735) -> (274.446, 144.392) construction
  line L6389 (274.446, 144.392) -> (274.6008, 144.4129) construction
  line L6390 (274.6008, 144.4129) -> (274.7555, 144.4359) construction
  line L6391 (274.7555, 144.4359) -> (274.9102, 144.461) construction
  line L6392 (274.9102, 144.461) -> (275.0649, 144.4879) construction
  line L6393 (275.0649, 144.4879) -> (275.2195, 144.5162) construction
  line L6394 (275.2195, 144.5162) -> (275.3741, 144.5458) construction
  line L6395 (275.3741, 144.5458) -> (275.5286, 144.5767) construction
  line L6396 (275.5286, 144.5767) -> (275.6831, 144.6087) construction
  line L6397 (275.6831, 144.6087) -> (275.8375, 144.6421) construction
  line L6398 (275.8375, 144.6421) -> (275.9918, 144.6768) construction
  line L6399 (275.9918, 144.6768) -> (276.146, 144.7129) construction
  line L6400 (276.146, 144.7129) -> (276.3002, 144.7503) construction
  line L6401 (276.3002, 144.7503) -> (276.4542, 144.7891) construction
  line L6402 (276.4542, 144.7891) -> (276.6082, 144.8291) construction
  line L6403 (276.6082, 144.8291) -> (276.7621, 144.8703) construction
  line L6404 (276.7621, 144.8703) -> (276.9159, 144.9127) construction
  line L6405 (276.9159, 144.9127) -> (277.0696, 144.9561) construction
  line L6406 (277.0696, 144.9561) -> (277.2232, 145.0007) construction
  line L6407 (277.2232, 145.0007) -> (277.3767, 145.0464) construction
  line L6408 (277.3767, 145.0464) -> (277.53, 145.0932) construction
  line L6409 (277.53, 145.0932) -> (277.6833, 145.1411) construction
  line L6410 (277.6833, 145.1411) -> (277.8364, 145.1901) construction
  line L6411 (277.8364, 145.1901) -> (277.9894, 145.2401) construction
  line L6412 (277.9894, 145.2401) -> (278.1423, 145.2913) construction
  line L6413 (278.1423, 145.2913) -> (278.2951, 145.3434) construction
  line L6414 (278.2951, 145.3434) -> (278.4478, 145.3965) construction
  line L6415 (278.4478, 145.3965) -> (278.6003, 145.4507) construction
  line L6416 (278.6003, 145.4507) -> (278.7526, 145.5058) construction
  line L6417 (278.7526, 145.5058) -> (278.9049, 145.562) construction
  line L6418 (278.9049, 145.562) -> (279.057, 145.619) construction
  line L6419 (279.057, 145.619) -> (279.209, 145.6771) construction
  line L6420 (279.209, 145.6771) -> (279.3608, 145.7361) construction
  line L6421 (279.3608, 145.7361) -> (279.5124, 145.7961) construction
  line L6422 (279.5124, 145.7961) -> (279.664, 145.857) construction
  line L6423 (279.664, 145.857) -> (279.8153, 145.9188) construction
  line L6424 (279.8153, 145.9188) -> (279.9665, 145.9815) construction
  line L6425 (279.9665, 145.9815) -> (280.1176, 146.0452) construction
  line L6426 (280.1176, 146.0452) -> (280.2685, 146.1097) construction
  line L6427 (280.2685, 146.1097) -> (280.4192, 146.1751) construction
  line L6428 (280.4192, 146.1751) -> (280.5698, 146.2415) construction
  line L6429 (280.5698, 146.2415) -> (280.7202, 146.3087) construction
  line L6430 (280.7202, 146.3087) -> (280.8704, 146.3767) construction
  line L6431 (280.8704, 146.3767) -> (281.0205, 146.4457) construction
  line L6432 (281.0205, 146.4457) -> (281.1704, 146.5154) construction
  line L6433 (281.1704, 146.5154) -> (281.3201, 146.5861) construction
  line L6434 (281.3201, 146.5861) -> (281.4696, 146.6575) construction
  line L6435 (281.4696, 146.6575) -> (281.619, 146.7299) construction
  line L6436 (281.619, 146.7299) -> (281.7682, 146.803) construction
  line L6437 (281.7682, 146.803) -> (281.9172, 146.877) construction
  line L6438 (281.9172, 146.877) -> (282.066, 146.9518) construction
  line L6439 (282.066, 146.9518) -> (282.2146, 147.0274) construction
  line L6440 (282.2146, 147.0274) -> (282.3631, 147.1038) construction
  line L6441 (282.3631, 147.1038) -> (282.5113, 147.181) construction
  line L6442 (282.5113, 147.181) -> (282.6594, 147.259) construction
  line L6443 (282.6594, 147.259) -> (282.8072, 147.3378) construction
  line L6444 (282.8072, 147.3378) -> (282.9549, 147.4174) construction
  line L6445 (282.9549, 147.4174) -> (283.1023, 147.4977) construction
  line L6446 (283.1023, 147.4977) -> (283.2496, 147.5789) construction
  line L6447 (283.2496, 147.5789) -> (283.3672, 147.6444) construction
  line L6448 (283.3672, 147.6444) -> (283.4554, 147.6939) construction
  line L6449 (283.4554, 147.6939) -> (283.5141, 147.7271) construction
  line L6450 (283.5141, 147.7271) -> (283.5435, 147.7437) construction
  arc A171 (161.0254, 119.7202) -> (161.7599, 122.4018) centre (160.0059, 121.4408) ccw
  arc A172 (155.6851, 193.8) -> (153.0327, 190.1492) centre (212.132, 150) ccw
  arc A173 (269.1057, 157.2806) -> (271.2762, 155.5428) centre (271.0895, 157.5341) ccw
  arc A174 (170.3188, 110.6216) -> (167.5414, 110.7517) centre (168.8628, 109.2504) ccw